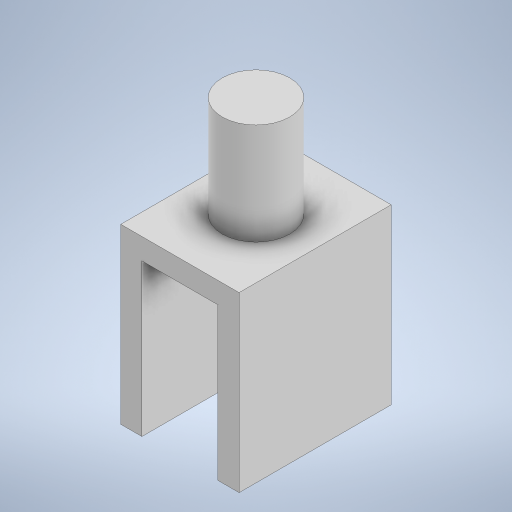
# Autodesk Inventor part: HUDSON 1-19-LEAFSPRING-AXLE BOX SADDLE
Saved by Autodesk Inventor 2024.2 (Build 282272000, 272)
## iProperties
Created: 2024-10-08
Part Number: HUDSON 1-19-LEAFSPRING-AXLE BOX SADDLE
Material: Generic
Document SubType Name: Modeling
Designer: Jimena Brenes
Density: 1 g/cm^3
Appearance: Default
Author: Jimena Brenes
Autodesk Inventor part; units mm, degrees
ref_plane "YZ Plane" through (0, 0, 0) normal (1, 0, 0) x (0, 1, 0)
ref_plane "XZ Plane" through (0, 0, 0) normal (0, 1, 0) x (-1, 0, 0)
ref_plane "XY Plane" through (0, 0, 0) normal (0, 0, 1) x (1, 0, 0)
sketch "Sketch1" plane through (0, 0, 0) normal (0, 0, 1) x (1, 0, 0)
  line L0 (0, 0) -> (0, 20.5)
  line L1 (0, 0) -> (2.5, 0)
  line L2 (2.5, 0) -> (2.5, 18)
  line L3 (2.5, 18) -> (11.5, 18)
  line L4 (11.5, 18) -> (11.5, 0)
  line L5 (11.5, 0) -> (14, 0)
  line L6 (0, 20.5) -> (14, 20.5)
  line L7 (14, 20.5) -> (14, 0)
  dimension "d0" = 20.5
  dimension "d1" = 2.5
  dimension "d2" = 18
  dimension "d3" = 9
  dimension "d4" = 2.5
  constraints: 16 end point, 4 perpendicular, 2 horizontal, 2 point on line, 1 vertical
  measures "d0" distance of L0.start L0.end
  measures "d1" distance of L0.start L1.end
  measures "d2" distance of L1.end L2.end
  measures "d3" distance of L2.end L3.end
  measures "d4" distance between parallel lines of L7 L4
extrude "Extrusion1" add sketch "Sketch1" against normal blind 18
sketch "Sketch2" plane through (0, 20.5, 0) normal (0, 1, 0) x (1, 0, 0)
  circle A0 centre (7, 9) radius 4
  line L0 (0, 0) -> (0, 18) projected
  line L1 (14, 0) -> (0, 0) projected
  dimension "d7" = 8
  dimension "d8" = 7
  dimension "d9" = 9
  constraints: 1 centre point
  measures "d7" diameter of A0
  measures "d8" distance from line of L0 A0.centre
  measures "d9" distance from line of L1 A0.centre
extrude "Extrusion2" add sketch "Sketch2" along normal blind 12
body "Solid1"
